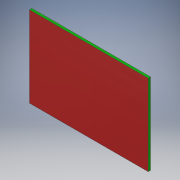
# Autodesk Inventor part: MainBoard
Saved by Autodesk Inventor 2019.3 (Build 233278000, 278)
## iProperties
Created: 2019-03-27
Part Number: MainBoard
Material: Generic
Document SubType Name: Modeling
Designer: Willist
Density: 1 g/cm^3
Appearance: Default
Author: Willist
Autodesk Inventor part; units mm, degrees
ref_plane "YZ Plane" through (0, 0, 0) normal (1, 0, 0) x (0, 1, 0)
ref_plane "XZ Plane" through (0, 0, 0) normal (0, 1, 0) x (-1, 0, 0)
ref_plane "XY Plane" through (0, 0, 0) normal (0, 0, 1) x (1, 0, 0)
sketch "Sketch1" plane through (0, 0, 0) normal (0, 0, 1) x (1, 0, 0)
  line L0 (-55, 37.5) -> (55, 37.5)
  line L1 (55, 37.5) -> (55, -37.5)
  line L2 (55, -37.5) -> (-55, -37.5)
  line L3 (-55, -37.5) -> (-55, 37.5)
  point P0 (0, 0)
  dimension "d0" = 110
  dimension "d1" = 75
  constraints: 8 end point, 2 parallel, 1 horizontal, 1 perpendicular
  measures "d0" distance of L1.end L2.end
  measures "d1" distance of L0.end L1.end
extrude "Extrusion1" add sketch "Sketch1" along normal blind 2.17
body "Solid1"
